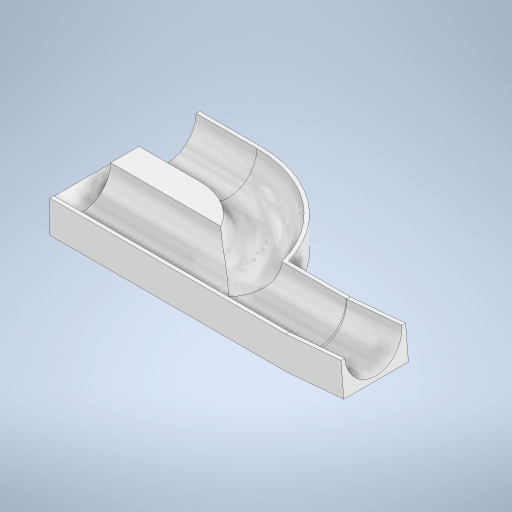
# Autodesk Inventor part: Libera todas
Saved by Autodesk Inventor 2024 (Build 280153000, 153)
## iProperties
Created: 2023-05-11
Part Number: Libera todas
Material: Plástico PET
Document SubType Name: Modeling
Designer: jpjoa
Density: 1.541 g/cm^3
Appearance: Branco
Author: jpjoa
Autodesk Inventor part; units mm, degrees
ref_plane "YZ Plane" through (0, 0, 0) normal (1, 0, 0) x (0, 1, 0)
ref_plane "XZ Plane" through (0, 0, 0) normal (0, 1, 0) x (-1, 0, 0)
sketch "Esboço1" plane through (0, 0, 0) normal (0, 1, 0) x (-1, 0, 0)
  line L0 (-1.2, -1.2) -> (-73.711, -1.2)
  line L1 (-73.711, -1.2) -> (-73.711, -19.2)
  line L2 (-1.2, -19.2) -> (-1.2, -1.2)
  line L3 (-1.2, -46.2) -> (-19.2, -46.2)
  line L4 (-1.2, -28.2) -> (-19.2, -28.2)
  arc A0 (-34.7885, -19.2) -> (-19.2, -28.2) centre (-19.2, -10.2) ccw
  line L5 (-19.2, -28.2) -> (-19.2, -10.2) construction
  line L6 (-34.7885, -19.2) -> (-19.2, -10.2) construction
  arc A1 (-54.0569, -19.2) -> (-19.2, -46.2) centre (-19.2, -10.2) ccw
  line L7 (-73.711, -19.2) -> (-54.0569, -19.2)
  line L8 (-34.7885, -19.2) -> (-1.2, -19.2)
  line L9 (-1.2, -28.2) -> (-1.2, -46.2)
  line L10 (0, -20.4) -> (0, 0)
  line L11 (0, 0) -> (-74.911, 0)
  line L12 (-74.911, 0) -> (-74.911, -20.4)
  line L13 (-74.911, -20.4) -> (-54.9743, -20.4)
  arc A2 (-54.9743, -20.4) -> (-19.2, -47.4) centre (-19.2, -10.2) ccw
  line L14 (-19.2, -47.4) -> (0, -47.4)
  line L15 (0, -47.4) -> (0, -27)
  line L16 (0, -27) -> (-19.2, -27)
  arc A3 (-32.5492, -20.4) -> (-19.2, -27) centre (-19.2, -10.2) ccw
  line L17 (-32.5492, -20.4) -> (0, -20.4)
  line L18 (-1.2, -19.2) -> (0, -19.2)
  line L19 (-1.2, -1.2) -> (0, -1.2)
  line L20 (-1.2, -28.2) -> (0, -28.2)
  line L21 (-1.2, -46.2) -> (0, -46.2)
  line L22 (-73.711, -19.2) -> (-74.911, -19.2)
  line L23 (-73.711, -1.2) -> (-74.911, -1.2)
  line L24 (0, -20.4) -> (0, -27)
  dimension "d1" = 60
  dimension "d2" = 18
  dimension "d3" = 18
  dimension "d4" = 18
  dimension "d5" = 1.2
  dimension "d7" = 18
  dimension "d8" = 74.911
  dimension "d47" = 9
  constraints: 50 end point, 15 perpendicular, 8 point on circle, 8 point on line, 4 centre point, 3 horizontal, 2 coincident, 2 horizontal alignment, 2 vertical alignment, 1 parallel, 1 tangent, 1 vertical, 9 other
  measures "d1" angle of L6 L5
  measures "d2" radial gap between concentric circles of A0 A1
  measures "d3" distance of L4.start L3.start
  measures "d4" distance of L2.start L0.start
  measures "d5" distance between parallel lines of L8 L17
  measures "d7" distance of L4.start L4.end
  measures "d8" distance of L10.end L11.end
  measures "d47" distance between parallel lines of L4 L8
extrude "Extrusão1" add sketch "Esboço1" against normal blind 1.2
extrude "Extrusão2" add sketch "Esboço1" along normal blind 9 contours L0 L23 L12 L11 L10 L19 | L18 L10 L17 A3 L16 L15 L20 L4 A0 L8 | L7 A1 L3 L21 L15 L14 A2 L13 L12 L22 | L24 L16 A3 L17
sketch "Esboço2" plane through (0, -1.2, 0) normal (0, -1, 0) x (1, 0, 0)
  line L0 (10, -37.2) -> (10, -10.2)
  line L1 (10, -10.2) -> (-10, -10.2)
  line L2 (-10, -10.2) -> (-10, -37.2)
  line L3 (-10, -37.2) -> (10, -37.2)
  line L4 (0, -46.2) -> (0, -28.2) projected
  line L5 (0, -19.2) -> (0, -1.2) projected
  point P0 (0, 0)
  point P1 (0, -10.2)
  point P2 (0, -37.2)
  point P3 (0, -37.2)
  point P4 (0, -10.2)
  dimension "d13" = 20
  constraints: 8 end point, 4 midpoint, 3 perpendicular, 2 coincident, 1 horizontal, 1 vertical alignment
  measures "d13" distance between parallel lines of L0 L2
extrude "Extrusão3" add sketch "Esboço2" along normal blind 2.4
fillet "Arredondamento1" radius 9 7 edges at (9.6, 0, -46.2) (41.2454, 0, -38.6605) (28.2, 0, -25.7885) (9.6, 0, -28.2) (17.3942, 0, -19.2) (64.4839, 0, -19.2) (37.4555, 0, -1.2)
sketch "Esboço3" plane through (0, -1.2, 0) normal (0, 0, 1) x (1, 0, 0)
  line L0 (74.911, 0) -> (92.8425, 1.5688)
  line L1 (74.911, 0) -> (0, 0) projected
  line L2 (74.4657, 10.2) -> (91.9535, 11.73)
  line L3 (91.9535, 11.73) -> (92.8425, 1.5688)
  line L4 (74.911, 0) -> (74.4657, 10.2)
  point P0 (0, 1.2)
  point P1 (74.911, 10.2)
  dimension "d18" = 5
  dimension "d19" = 10.2
  dimension "d20" = 18
  constraints: 8 end point, 2 coincident, 1 horizontal alignment, 1 parallel, 1 perpendicular
  measures "d18" angle of L1 L0
  measures "d19" distance between parallel lines of L0 L2
  measures "d20" distance of L0.start L0.end
extrude "Extrusão4" add sketch "Esboço3" against normal up to surface (20.4 mm away)
ref_plane "Plano de trabalho1" through (54.9743, -1.2, -10.2) normal (0, 0, -1) x (-1, 0, 0)
sketch "Esboço4" plane through (54.9743, -1.2, -10.2) normal (0, 0, -1) x (-1, 0, 0)
  line L0 (-36.9792, 11.73) -> (-19.4914, 10.2)
  line L1 (-36.9792, 11.73) -> (-19.4914, 10.2) projected
  line L2 (-37.7636, 2.7642) -> (-19.8843, 1.2)
  line L3 (54.9743, 1.2) -> (-19.8843, 1.2) projected
  line L4 (-19.4914, 10.2) -> (-19.8843, 1.2) projected
  line L5 (-36.9792, 11.73) -> (-37.7636, 2.7642)
  line L6 (-19.8843, 1.2) -> (-19.4914, 10.2)
  point P0 (54.9743, 1.2)
  point P1 (-19.8843, 1.2)
  dimension "d23" = 9
  constraints: 8 end point, 4 coincident, 1 collinear, 1 parallel, 1 perpendicular
  measures "d23" distance between parallel lines of L0 L2
extrude "Extrusão5" cut sketch "Esboço4" along normal mid plane 18
fillet "Arredondamento2" radius 9 2 edges at (83.7983, 0.7821, -19.2) (83.7983, 0.7821, -1.2)
fillet_without_effect "Arredondamento3"
sketch "Esboço5" plane through (0, -1.2, 0) normal (0, -1, 0) x (1, 0, 0)
  line L0 (11.8217, -9) -> (11.8217, -11.4)
  line L1 (11.8217, -11.4) -> (19.6217, -11.4)
  line L2 (19.6217, -11.4) -> (19.6217, -9)
  line L3 (19.6217, -9) -> (11.8217, -9)
  line L4 (47.0437, -9) -> (47.0437, -11.4)
  line L5 (47.0437, -11.4) -> (54.8437, -11.4)
  line L6 (54.8437, -11.4) -> (54.8437, -9)
  line L7 (54.8437, -9) -> (47.0437, -9)
  line L8 (0, 0) -> (0, -10.2) projected
  line L9 (74.4657, -1.2) -> (74.4657, -19.2) projected
  line L10 (92.8425, 0) -> (92.8425, -20.4) projected
  line L11 (74.911, -20.4) -> (74.911, 0) projected
  point P0 (19.6217, -10.2)
  point P1 (47.0437, -10.2)
  point P2 (11.8217, -10.2)
  point P3 (92.8425, -10.2)
  dimension "d28" = 7.8
  dimension "d29" = 2.4
  dimension "d31" = 27.422
  dimension "d46" = 19.622
  constraints: 16 end point, 6 perpendicular, 4 midpoint, 2 equal length, 2 horizontal alignment, 2 vertical
  measures "d28" distance of L0.end L1.end
  measures "d29" distance of L1.end L2.end
  measures "d31" distance between parallel lines of L4 L2
  measures "d46" distance between parallel lines of L9 L6
extrude "Extrusão6" add sketch "Esboço5" along normal blind 5.4
sketch "Esboço6" plane through (11.8217, -1.2, -9) normal (0, 0, 1) x (1, 0, 0)
  circle A0 centre (3.9, -2.7) radius 1.5
  circle A1 centre (3.9, -2.7) radius 2.7
  line L0 (6.6, -2.7) -> (6.6, -1.2)
  line L1 (63.0893, 0) -> (-11.8217, 0) projected
  line L2 (7.8, -5.4) -> (0, -5.4) projected
  line L3 (1.2, -2.7) -> (1.2, -1.2)
  line L4 (0, 0) -> (7.8, 0) projected
  line L5 (0, 0) -> (0, 0)
  line L6 (0, 0) -> (0, -5.4) projected
  line L7 (0, 0) -> (0, -5.4)
  line L8 (0, -5.4) -> (7.8, -5.4)
  line L9 (7.8, -5.4) -> (7.8, 0)
  line L10 (7.8, 0) -> (7.8, 0)
  arc A2 (7.8, 0) -> (6.6, -1.2) centre (7.8, -1.2) ccw
  arc A3 (1.2, -1.2) -> (0, 0) centre (0, -1.2) ccw
  circle A4 centre (39.122, -2.7) radius 1.5
  circle A5 centre (39.122, -2.7) radius 2.7
  line L11 (41.822, -2.7) -> (41.822, -1.2)
  line L12 (36.422, -2.7) -> (36.422, -1.2)
  line L13 (43.022, -5.4) -> (35.222, -5.4) projected
  line L14 (43.022, 0) -> (43.022, -5.4) projected
  line L15 (35.222, -5.4) -> (43.022, -5.4) projected
  line L16 (43.022, -5.4) -> (35.222, -5.4)
  line L17 (43.022, 0) -> (35.222, 0) projected
  line L18 (35.222, -5.4) -> (35.222, 0)
  line L19 (35.222, 0) -> (35.222, 0)
  line L20 (43.022, -5.4) -> (43.022, 0)
  arc A6 (36.422, -1.2) -> (35.222, 0) centre (35.222, -1.2) ccw
  line L21 (43.022, 0) -> (43.022, 0)
  arc A7 (43.022, 0) -> (41.822, -1.2) centre (43.022, -1.2) ccw
  point P0 (-11.8217, 1.2)
  point P1 (6.6, 0)
  point P2 (3.9, -5.4)
  point P3 (1.2, 0)
  point P4 (41.822, 0)
  point P5 (36.422, 0)
  point P6 (39.122, -5.4)
  point P7 (3.9, -5.4)
  point P8 (35.222, 0)
  point P9 (39.122, -5.4)
  point P10 (43.022, 0)
  dimension "d35" = 3
  dimension "d36" = 1.2
  dimension "d37" = 2.7
  dimension "d38" = 1.2
  dimension "d39" = 3
  dimension "d40" = 1.2
  dimension "d41" = 1.2
  dimension "d42" = 1.2
  constraints: 28 end point, 12 point on circle, 12 tangent, 8 centre point, 8 point on line, 5 perpendicular, 4 vertical, 2 collinear, 2 horizontal, 2 midpoint, 2 vertical alignment, 1 equal radius, 1 horizontal alignment, 7 other
  measures "d35" diameter of A0
  measures "d36" radial gap between concentric circles of A0 A1
  measures "d38" radius of A2
  measures "d39" diameter of A4
  measures "d40" radial gap between concentric circles of A4 A5
  measures "d41" radius of A6
  measures "d42" radius of A7
extrude "Extrusão7" cut sketch "Esboço6" against normal up to surface (2.4 mm away) contours A0 | L0 A2 L9 L2 A1 | L2 L6 A3 L3 A1 | L14 L13 A5 L11 A7 | A6 L12 A5 L13 L18 | A4
equation "\"d3\" = Diâmetro_esfera"
equation "\"d4\" = Diâmetro_esfera"
equation "\"d5\" = Margem"
equation "\"d7\" = Diâmetro_esfera"
equation "\"d8\" = Distância_fim"
equation "\"d47\" = Espessura_entre_trilhos"
equation "\"d9\" = Margem"
equation "\"d11\" = 0.5 * Diâmetro_esfera"
equation "\"d14\" = 2 * Margem"
equation "\"d16\" = 0.5 * Diâmetro_esfera"
equation "\"d19\" = 0.5 * Diâmetro_esfera + Margem"
equation "\"d20\" = Diâmetro_esfera"
equation "\"d21\" = 2 * Margem"
equation "\"d23\" = 0.5 * Diâmetro_esfera"
equation "\"d24\" = Diâmetro_esfera"
equation "\"d26\" = 0.5 * Diâmetro_esfera"
equation "\"d27\" = 0.5 * Diâmetro_esfera"
equation "\"d28\" = Parafuso + 4 * Margem"
equation "\"d29\" = 2 * Margem"
equation "\"d31\" = Distância_parafuso"
equation "\"d46\" = Distância_parafuso_fim"
equation "\"d33\" = Parafuso + 2 * Margem"
equation "\"d35\" = Parafuso"
equation "\"d36\" = Margem"
equation "\"d37\" = 0.5 * Parafuso + Margem"
equation "\"d39\" = Parafuso"
equation "\"d40\" = Margem"
equation "\"d43\" = Parafuso + 2 * Margem"
equation "\"Diâmetro_esfera\" = 18"
equation "\"Filamento\" = 0.4"
equation "\"Margem\" = 3 * Filamento"
equation "\"Espessura_entre_trilhos\" = 9"
equation "\"Distância_fim\" = 74.911"
equation "\"Parafuso\" = 3"
equation "\"Distância_parafuso\" = 27.422"
equation "\"Distância_parafuso_fim\" = 19.622"
